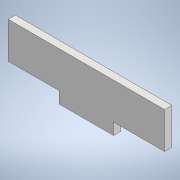
# Autodesk Inventor part: lead_2
Saved by Autodesk Inventor 2022 (Build 260153000, 153)
## iProperties
Created: 2022-12-25
Part Number: lead_2
Material: Lead
Document SubType Name: Modeling
Designer: Kamil
Mass: 130.092 g
Surface Area: 51.728 cm^2
Volume: 11.472 cm^3
Density: 11.34 g/cm^3
Appearance: Lead
Author: Kamil
Autodesk Inventor part; units mm, degrees
ref_plane "YZ Plane" through (0, 0, 0) normal (1, 0, 0) x (0, 1, 0)
ref_plane "XZ Plane" through (0, 0, 0) normal (0, 1, 0) x (-1, 0, 0)
ref_plane "XY Plane" through (0, 0, 0) normal (0, 0, 1) x (1, 0, 0)
sketch "Sketch1" plane through (0, 0, 0) normal (0, 0, 1) x (1, 0, 0)
  circle A0 centre (0, -3.2) radius 2.6186 projected
  line L0 (-15, 15.4) -> (-15, -13.4) projected
  arc A1 (-15, -13.4) -> (-13, -15.4) centre (-13, -13.4) ccw projected
  line L1 (-13, -15.4) -> (13, -15.4) projected
  arc A2 (13, -15.4) -> (15, -13.4) centre (13, -13.4) ccw projected
  line L2 (15, -13.4) -> (15, 15.4) projected
  line L3 (15, 15.4) -> (48, 15.4) projected
  line L4 (48, 15.4) -> (48, 80.7) projected
  line L5 (48, 80.7) -> (-48, 80.7) projected
  line L6 (-48, 80.7) -> (-48, 15.4) projected
  line L7 (-48, 15.4) -> (-15, 15.4) projected
  circle A3 centre (-7.5, 5.8) radius 1.75 projected
  circle A4 centre (7.5, 5.8) radius 1.75 projected
  circle A5 centre (-7.5, -12.2) radius 1.75 projected
  circle A6 centre (7.5, -12.2) radius 1.75 projected
  line L8 (-5.6525, 9) -> (5.6525, 9) projected
  circle A7 centre (0, -3.2) radius 2.6186 projected
  arc A8 (15, 7) -> (13, 9) centre (13, 7) ccw projected
  line L9 (9.3475, 9) -> (13, 9) projected
  line L10 (11.195, 5.8) -> (9.3475, 9) projected
  line L11 (9.3475, 2.6) -> (11.195, 5.8) projected
  line L12 (5.6525, 2.6) -> (9.3475, 2.6) projected
  line L13 (3.805, 5.8) -> (5.6525, 2.6) projected
  line L14 (5.6525, 9) -> (3.805, 5.8) projected
  line L15 (-5.6525, 9) -> (5.6525, 9) projected
  line L16 (-5.6525, 9) -> (-3.805, 5.8) projected
  line L17 (-3.805, 5.8) -> (-5.6525, 2.6) projected
  line L18 (-5.6525, 2.6) -> (-9.3475, 2.6) projected
  line L19 (-9.3475, 2.6) -> (-11.195, 5.8) projected
  line L20 (-11.195, 5.8) -> (-9.3475, 9) projected
  line L21 (-9.3475, 9) -> (-13, 9) projected
  arc A9 (-13, 9) -> (-15, 7) centre (-13, 7) ccw projected
  line L22 (-15, 7) -> (-15, -13.4) projected
  arc A10 (-15, -13.4) -> (-13, -15.4) centre (-13, -13.4) ccw projected
  line L23 (-13, -15.4) -> (-9.3475, -15.4) projected
  line L24 (-9.3475, -15.4) -> (-11.195, -12.2) projected
  line L25 (-11.195, -12.2) -> (-9.3475, -9) projected
  line L26 (-9.3475, -9) -> (-5.6525, -9) projected
  line L27 (-5.6525, -9) -> (-3.805, -12.2) projected
  line L28 (-3.805, -12.2) -> (-5.6525, -15.4) projected
  line L29 (-5.6525, -15.4) -> (5.6525, -15.4) projected
  line L30 (3.805, -12.2) -> (5.6525, -15.4) projected
  line L31 (5.6525, -9) -> (3.805, -12.2) projected
  line L32 (9.3475, -9) -> (5.6525, -9) projected
  line L33 (11.195, -12.2) -> (9.3475, -9) projected
  line L34 (9.3475, -15.4) -> (11.195, -12.2) projected
  line L35 (13, -15.4) -> (9.3475, -15.4) projected
  arc A11 (13, -15.4) -> (15, -13.4) centre (13, -13.4) ccw projected
  line L36 (15, 7) -> (15, -13.4) projected
  line L37 (5.6525, 9) -> (9.3475, 9) projected
  line L38 (-5.6525, 9) -> (-9.3475, 9) projected
  line L39 (48, 15.4) -> (43, 15.4)
  line L40 (43, 15.4) -> (43, 80.7)
  line L41 (43, 80.7) -> (48, 80.7)
  line L42 (48, 80.7) -> (48, 15.4)
  line L43 (-48, 15.4) -> (-43, 15.4)
  line L44 (-43, 15.4) -> (-43, 80.7)
  line L45 (-43, 80.7) -> (-48, 80.7)
  line L46 (-48, 80.7) -> (-48, 15.4)
  line L47 (43, 15.4) -> (-43, 15.4)
  line L48 (-43, 15.4) -> (-43, 35.4)
  line L49 (-43, 35.4) -> (43, 35.4)
  line L50 (43, 35.4) -> (43, 15.4)
  line L51 (15, 9) -> (-15, 9)
  point P0 (0, 0)
  point P1 (13, 9)
  point P2 (43, 35.4)
  dimension "d0" = 5
  dimension "d1" = 5
  dimension "d2" = 20
  constraints: 26 end point, 6 parallel, 5 point on line, 4 perpendicular, 3 horizontal
  measures "d0" distance of L40.end L41.end
  measures "d1" distance of L45.end L44.end
  measures "d2" distance of L47.end L48.end
extrude "Extrusion1" add sketch "Sketch1" along normal blind 6 contours L47 L2 L51 L9 L37 L8 L38 L21 L0 | L7 L44 L49 L40 L3 L47
body "Solid1"
